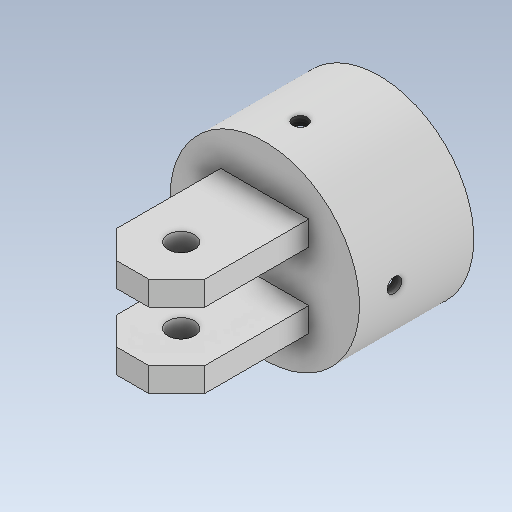
# Autodesk Inventor part: polar_axle
Saved by Autodesk Inventor 2021 (Build 250183000, 183)
## iProperties
Created: 2023-11-16
Part Number: polar_axle
Material: Generic
Document SubType Name: Modeling
Designer: vtoth
Density: 1 g/cm^3
Appearance: Default
d0: 1,000 ul
d1: 4,000 mm
d3: 52,000 mm
d5: 40,000 mm
d6: 60,000 mm
d7: 38,000 mm
d8: 18,000 mm
d9: 45,000 mm
d11: 45,000 mm
d12: 0,00 deg
d13: 23,000 mm
d14: 0,00 deg
tav: 23,000 mm
d17: 78,000 mm
Author: vtoth
Autodesk Inventor part; units mm, degrees
ref_plane "YZ Plane" through (0, 0, 0) normal (1, 0, 0) x (0, 1, 0)
ref_plane "XZ Plane" through (0, 0, 0) normal (0, 1, 0) x (-1, 0, 0)
ref_plane "XY Plane" through (0, 0, 0) normal (0, 0, 1) x (1, 0, 0)
derived "skeleton_1.ipt"
sketch "Sketch1" plane through (0, 0, 0) normal (0, 1, 0) x (-1, 0, 0)
  line L0 (0, 0) -> (0, 550)
  circle A0 centre (0, 550) radius 6
  line L1 (0, 550) -> (43.8812, 590.9199)
  line L2 (-15.7936, 654.9134) -> (83.0961, 548.8671)
  line L3 (111.4949, 533.0759) -> (80.291, 566.538)
  line L4 (96.8679, 519.4359) -> (65.6639, 552.898)
  line L5 (0, 0) -> (-350, 0)
  line L6 (11.0017, 632.044) -> (5.1509, 626.588)
  point P0 (0, 440)
sketch "Sketch2" plane through (15.7936, 0, 654.9134) normal (-0.6819984, 0, -0.7313537) x (0, -1, 0)
  line L0 (0, -60) -> (0, 0) construction
  line L1 (-69.5467, -18.635) -> (77.2741, 20.7055)
  circle A0 centre (0, 0) radius 10
  line L2 (20.1846, -4.9443) -> (20.2151, -4.9361)
  line L3 (-20.2054, 4.9388) -> (-20.1742, 4.9471)
  line L4 (69.2185, 23.7234) -> (71.8067, 14.0642)
  point P0 (0, 0)
  point P1 (0, 0)
  point P2 (0, 0)
  point P3 (0, 10)
  point P4 (0, 10)
  point P5 (0, 10)
  point P6 (-55.0578, -14.7527)
  point P7 (43.4667, 11.6469)
sketch "Sketch3" plane through (0.6506, -77.2741, 669.0345) normal (-0.1892883, -0.9659258, 0.1765142) x (0.9813346, -0.1923079, 0)
  line L0 (0, 0) -> (-97.0439, -107.738) construction
  line L1 (71.5956, -76.8054) -> (-71.5956, 76.8054)
  circle A0 centre (0, 0) radius 6
  line L2 (36.574, 34.0931) -> (-36.574, -34.0931)
  line L3 (-130.114, 22.2564) -> (-13.0771, 131.3544)
  point P0 (0, 0)
  point P1 (0, 0)
  point P2 (0, 0)
  point P3 (0, 0)
  point P4 (-70.6912, 42.1041)
ref_plane "Work Plane1" through (15.7936, 0, 654.9134) normal (-0.6819984, 0, -0.7313537) x (0, -1, 0)
ref_plane "Work Plane2" through (0.6506, -77.2741, 669.0345) normal (-0.1892883, -0.9659258, 0.1765142) x (0.9813346, -0.1923079, 0)
sketch "Sketch4" plane through (0, 0, 0) normal (0, 1, 0) x (-1, 0, 0)
  circle A0 centre (0, 550) radius 6 projected
  line L0 (0, 0) -> (0, 550) projected
  line L1 (-43, 460) -> (-43, 512)
  line L2 (-43, 512) -> (43, 512)
  line L3 (43, 512) -> (43, 460)
  line L4 (43, 460) -> (39, 460)
  line L5 (39, 460) -> (39, 505)
  line L6 (-39, 505) -> (-39, 460)
  line L7 (-39, 460) -> (-43, 460)
  line L8 (-20, 512) -> (-20, 559.2721)
  line L9 (-20, 559.2721) -> (-7.2721, 572)
  line L10 (-7.2721, 572) -> (7.2721, 572)
  line L11 (7.2721, 572) -> (20, 559.2721)
  line L12 (20, 559.2721) -> (20, 512)
  line L13 (39, 505) -> (0, 505)
  line L14 (0, 512) -> (0, 505)
  line L15 (0, 505) -> (-39, 505)
  point P0 (0, 512)
  dimension "d1" = 4
  dimension "d3" = 52
  dimension "d5" = 40
  dimension "d6" = 60
  dimension "d7" = 38
  dimension "d8" = 18
  dimension "d9" = 45
  dimension "d17" = 78
  constraints: 30 end point, 10 perpendicular, 7 symmetric about line, 4 point on line, 1 collinear, 1 midpoint, 1 vertical
  measures "d1" distance between parallel lines of L3 L5
  measures "d3" distance between parallel lines of L2 L4
  measures "d5" distance between parallel lines of L12 L8
  measures "d6" distance between parallel lines of L2 L10
  measures "d7" distance from line of L2 A0.centre
  measures "d8" distance of L8.end L9.end
  measures "d9" distance between parallel lines of L4 L13
  measures "d17" diameter of L6 L0
revolve "Revolution1" add sketch "Sketch4" angle 360 about axis through (0, 0, 0) along (0, 0, 1) contours L0 L2 L3 L4 L5 L13
extrude "Extrusion1" add sketch "Sketch4" along normal mid plane 45 contours L2 L8 L9 L10 L11 L12
extrude "Extrusion2" cut sketch "Sketch4" along normal mid plane 23 contours L2 L8 L9 L10 L11 L12
ref_plane "Work Plane3" through (-43, 0, 512) normal (-1, 0, 0) x (0, -1, 0)
sketch "Sketch6" plane through (-43, 0, 512) normal (-1, 0, 0) x (0, -1, 0)
  line L0 (0, 0) -> (0, -52) construction
  line L1 (-43, -52) -> (43, -52) construction
  point P0 (0, -512)
  point P1 (0, -16)
  dimension "d18" = 36
  constraints: 1 point on line
  measures "d18" distance from line of L1 point (0, -16)
hole "Hole1" at (-43, 0, 496) direction (1, 0, 0) diameter 6.647 end up to face face through (0, 0, 482.5) facing (0, 0, -1) round with radius 39 far side no thread size "M8x1.25" class "6H" standard "ISO Metric profile"
pattern_circular "Circular Pattern1" count 4 over 360 about axis through (0, 0, 486) along (0, 0, -1) of "Hole1"
